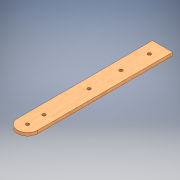
# Autodesk Inventor part: Część1
Saved by Autodesk Inventor 2017 (Build 210142000, 142)
## iProperties
Created: 2017-05-11
Part Number: Część1
Material: Drewno (wiśnia)
Document SubType Name: Modeling
Designer: Damian
Density: 0.63 g/cm^3
Appearance: Wiśnia — naturalna — niski połysk
Author: Damian
Autodesk Inventor part; units mm, degrees
ref_plane "YZ Plane" through (0, 0, 0) normal (1, 0, 0) x (0, 1, 0)
ref_plane "XZ Plane" through (0, 0, 0) normal (0, 1, 0) x (-1, 0, 0)
ref_plane "XY Plane" through (0, 0, 0) normal (0, 0, 1) x (1, 0, 0)
sketch "Szkic1" plane through (0, 0, 0) normal (0, 0, 1) x (1, 0, 0)
  line L0 (-10, 0) -> (-10, 0)
  line L1 (-20, 10) -> (-20, 143)
  line L2 (-20, 143) -> (0, 143)
  line L3 (0, 143) -> (0, 10)
  arc A0 (-20, 10) -> (-10, 0) centre (-10, 10) ccw
  arc A1 (-10, 0) -> (0, 10) centre (-10, 10) ccw
  circle A2 centre (-10, 10) radius 1.6
  circle A3 centre (-10, 26.143) radius 1.6
  circle A4 centre (-10, 70.581) radius 1.6
  circle A5 centre (-10, 102) radius 1.6
  point P0 (0, 0)
  point P1 (-20, 0)
  dimension "d0" = 20
  dimension "d1" = 143
  dimension "d2" = 10
  dimension "d3" = 3.2
  dimension "d4" = 16.143
  dimension "d5" = 3.2
  dimension "d6" = 60.581
  dimension "d7" = 3.2
  dimension "d8" = 102
  dimension "d9" = 3.2
  constraints: 8 end point, 6 centre point, 4 coincident, 4 point on circle, 4 point on line, 4 tangent, 2 parallel, 1 concentric, 1 horizontal, 1 perpendicular
  measures "d0" distance of L1.end L2.end
  measures "d1" distance of point (-20, 0) L1.end
  measures "d2" radius of A0
  measures "d3" diameter of A2
  measures "d4" distance of point (-10, 26.143) A1.centre
  measures "d5" diameter of A3
  measures "d6" distance of point (-10, 70.581) A0.centre
  measures "d7" diameter of A4
  measures "d8" distance of L0.end point (-10, 102)
  measures "d9" diameter of A5
extrude "Wyciągnięcie proste1" add sketch "Szkic1" along normal blind 3
sketch "Szkic2" plane through (0, 0, 3) normal (0, 0, 1) x (1, 0, 0)
  line L0 (0, 143) -> (-20, 143) projected
  point P0 (0, 0)
  point P1 (-10, 130)
  dimension "d12" = 13
  measures "d12" distance from line of point (-10, 130) L0
hole "Otwór1" at (-10, 130, 3) direction (0, 0, -1) diameter 3.2 end through all
